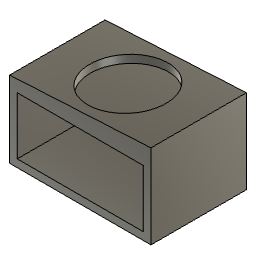
mac holder (Autodesk Fusion 360 design; units mm, degrees)
Autodesk Fusion 360 part; units mm, degrees
note: some values were not read from the file. Set by a fixed rule: which sketch regions a step uses.
sketch "Sketch1" plane through (0, 0, 0) normal (0, 0, 1) x (1, 0, 0)
  line L0 (0, 0) -> (37, 0)
  line L1 (37, 0) -> (37, 25)
  line L2 (37, 25) -> (0, 25)
  line L3 (0, 25) -> (0, 0)
  dimension "d1" = 37
  dimension "d2" = 25
  constraint horizontal L0
  constraint vertical L1
  constraint horizontal L2
  constraint vertical L3
  constraint coincident L0.start L3.end
  measures "d1" distance of L0.start L0.end
  measures "d2" distance of L0.start L2.end
extrude "Extrude1" add sketch "Sketch1" along normal blind 2
sketch "Sketch2" plane through (0, 0, 2) normal (0, 0, 1) x (-1, 0, 0)
  line L0 (0, -25) -> (0, 0)
  line L1 (0, 0) -> (-37, 0)
  line L2 (-37, 0) -> (-37, -25)
  line L3 (-37, -25) -> (0, -25)
  line L4 (0, -25) -> (-2, -25)
  line L5 (-2, -25) -> (-2, 0)
  line L6 (-2, 0) -> (0, 0)
  line L7 (0, 0) -> (0, -25)
  line L8 (-37, -25) -> (-35, -25)
  line L9 (-35, -25) -> (-35, 0)
  line L10 (-35, 0) -> (-37, 0)
  line L11 (-37, 0) -> (-37, -25)
  dimension "d5" = 2
  dimension "d6" = 25
  dimension "d7" = 2
  dimension "d8" = 25
  constraint horizontal L4
  constraint vertical L5
  constraint horizontal L6
  constraint vertical L7
  constraint coincident L0.start L3.end
  constraint horizontal L8
  constraint vertical L9
  constraint horizontal L10
  constraint vertical L11
  constraint coincident L2.end L3.start
  measures "d5" distance of L0.start L4.end
  measures "d6" distance of L0.start L0.end
  measures "d7" distance of L2.end L8.end
  measures "d8" distance of L2.end L1.end
extrude "Extrude2" add sketch "Sketch2" along normal blind 16 contours L0 L1 L3 L4 L5 L6 L7 | L1 L2 L3 L8 L9 L10 L11
sketch "Sketch3" plane through (0, 0, 18) normal (0, 0, 1) x (-1, 0, 0)
  line L0 (-37, 0) -> (-37, -25)
  line L1 (-37, -25) -> (-35, -25)
  line L2 (-35, -25) -> (-35, 0)
  line L3 (-35, 0) -> (-37, 0)
  line L4 (0, -25) -> (-37, -25)
  line L5 (-37, -25) -> (-37, 0)
  line L6 (-37, 0) -> (0, 0)
  line L7 (0, 0) -> (0, -25)
  constraint horizontal L4
  constraint vertical L5
  constraint horizontal L6
  constraint vertical L7
  constraint coincident L0.start L3.end
extrude "Extrude3" add sketch "Sketch3" along normal blind 20
sketch "Sketch4" plane through (0, 0, 0) normal (0, -1, 0) x (1, 0, 0)
  line L0 (0, 38) -> (0, 0)
  line L1 (0, 0) -> (37, 0)
  line L2 (37, 0) -> (37, 38)
  line L3 (37, 38) -> (0, 38)
  line L4 (2, 18) -> (35, 18)
  line L5 (35, 18) -> (35, 2)
  line L6 (35, 2) -> (2, 2)
  line L7 (2, 2) -> (2, 18)
  line L8 (0, 20) -> (37, 22)
  constraint coincident L0 L8.start
  constraint coincident L2 L8.end
extrude "Extrude4" cut sketch "Sketch4" against normal blind 40 contours L0 L2 L3 L8
sketch "Sketch5" plane through (-1.0779, 0, 19.9417) normal (-0.053975, 0, 0.998542) x (0, -1, 0)
  line L0 (-25, 38.1335) -> (-25, 1.0795)
  line L1 (-25, 1.0795) -> (0, 1.0795)
  line L2 (0, 1.0795) -> (0, 38.1335)
  line L3 (0, 38.1335) -> (-25, 38.1335)
  line L4 (-25, 1.0795) -> (-12.5, 1.0795)
  line L5 (-12.5, 1.0795) -> (-12.5, 19.5795)
  line L6 (-12.5, 19.5795) -> (-25, 19.5795)
  line L7 (-25, 19.5795) -> (-25, 1.0795)
  circle A0 centre (-12.5, 19.5795) radius 10
  dimension "d15" = 12.5
  dimension "d16" = 18.5
  dimension "d17" = 20
  constraint horizontal L4
  constraint vertical L5
  constraint horizontal L6
  constraint vertical L7
  constraint coincident L0.end L1.start
  constraint coincident L5.end L6.start
  measures "d15" distance of L0.end L4.end
  measures "d16" distance of L0.end L6.end
  measures "d17" diameter of A0
extrude "Extrude5" cut sketch "Sketch5" against normal blind 2 contours L5 L6 A0 | L5 L6 A0
extrude "Extrude6" add 1 faces at (24, 8.3333, 18) along direction (0, 0, -1) blind 1
